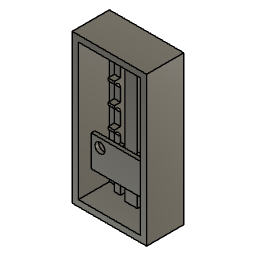
Progetto locker v3 (Autodesk Fusion 360 design; units mm, degrees)
Autodesk Fusion 360 part; units mm, degrees
note: some values were not read from the file. Chosen so that the rebuilt part matches the saved one: where a step ends.
sketch "Schizzo1" plane through (0, 0, 0) normal (0, 1, 0) x (1, 0, 0) in component "Scatola di fissaggio"
  line L0 (-30, -60) -> (30, -60)
  line L1 (30, -60) -> (30, 60)
  line L2 (30, 60) -> (-30, 60)
  line L3 (-30, 60) -> (-30, -60)
  point P0 (0, -60)
  point P1 (-30, 0)
  dimension "d1" = 60
  dimension "d2" = 120
  constraint horizontal L0
  constraint vertical L1
  constraint horizontal L2
  constraint vertical L3
  constraint midpoint L0 P0
  constraint midpoint L3 P1
  constraint vertical origin P0
  constraint horizontal origin P1
  measures "d1" distance of L0.start L0.end
  measures "d2" distance of L0.start L2.end
extrude "Estrusione1" add sketch "Schizzo1" along normal blind 30 makes body 1 in component "Scatola di fissaggio"
shell "Svuotamento1" thickness 5 removed faces 1 at (-10, 0, 20) on bodies 1 in component "Scatola di fissaggio"
ref_plane "Piano di lavoro1" through (0, 12.5, -55) normal (0, 0, 1) x (1, 0, 0) in component "Guida lineare"
sketch "Schizzo1 (2)" plane through (0, 12.5, -55) normal (0, 0, 1) x (1, 0, 0) in component "Guida lineare"
  line L0 (0, -21.6959) -> (0, 27.9147) construction
  line L1 (0, 5) -> (-5, 5)
  line L2 (-5, 5) -> (-5, 8.5)
  line L3 (-3.5, 10) -> (-2.5, 10)
  line L4 (-2.5, 10) -> (-2.5, 12.5)
  line L5 (25, 12.5) -> (-25, 12.5)
  line L6 (-5, 8.5) -> (-3.5, 10)
  line L7 (0, 5) -> (5, 5)
  line L8 (5, 5) -> (5, 8.5)
  line L9 (5, 8.5) -> (3.5, 10)
  line L10 (3.5, 10) -> (2.5, 10)
  line L11 (2.5, 10) -> (2.5, 12.5)
  point P0 (-5, 10)
  dimension "d7" = 2.5
  dimension "d8" = 5
  dimension "d9" = 5
  dimension "d10" = 2.5
  dimension "d11" = 1.5
  dimension "d12" = 1.5
  constraint vertical L0
  constraint coincident origin L0
  constraint coincident L0 L1.start
  constraint perpendicular L0 L1
  constraint perpendicular L1 L2
  constraint perpendicular L2 L3
  constraint perpendicular L3 L4
  constraint coincident L4.end L5
  constraint coincident P0 L2
  constraint coincident P0 L3
  constraint symmetric L0 L1.start L7.start
  constraint symmetric L0 L1.end L7.end
  constraint symmetric L0 L3.end L10.end
  constraint symmetric L0 L4.end L11.end
  constraint symmetric L0 L2.end L8.end
  constraint symmetric L0 L3.start L9.end
  measures "d7" distance of L3.end L4.end
  measures "d8" distance of L1.end P0
  measures "d9" distance of L1.start L1.end
  measures "d10" distance of L0 L4
  measures "d11" distance of P0 L2.end
  measures "d12" distance of P0 L3.start
extrude "Estrusione1'" add sketch "Schizzo1 (2)" along normal blind 110 separate body makes body 2 in component "Guida lineare"
sketch "Schizzo5" plane through (0, 0, 0) normal (0, 0, 1) x (1, 0, 0) in component "Base mobile"
  line L0 (5, 21) -> (3.5, 22.5)
  line L1 (5, 17.5) -> (5, 21)
  line L2 (0, 17.5) -> (5, 17.5)
  line L3 (0, 17) -> (5.5, 17)
  line L4 (5.5, 17) -> (5.5, 21.2071)
  line L5 (5.5, 21.2071) -> (3.8536, 22.8536)
  line L6 (3.8536, 22.8536) -> (8.8536, 22.8536)
  line L7 (8.8536, 22.8536) -> (8.8536, 12.8536)
  line L8 (8.8536, 12.8536) -> (0, 12.8536)
  line L9 (0, -9.1959) -> (0, 40.4147)
  line L10 (-8.8536, 12.8536) -> (0, 12.8536)
  line L11 (-8.8536, 22.8536) -> (-8.8536, 12.8536)
  line L12 (0, 17) -> (-5.5, 17)
  line L13 (-5.5, 17) -> (-5.5, 21.2071)
  line L14 (-3.8536, 22.8536) -> (-8.8536, 22.8536)
  line L15 (-5.5, 21.2071) -> (-3.8536, 22.8536)
  dimension "d24" = 0.5
  dimension "d25" = 10
  dimension "d26" = 5
  constraint perpendicular L1 L6
  constraint perpendicular L6 L7
  constraint perpendicular L7 L8
  constraint coincident L8.end L9
  constraint symmetric L3.start L9 L12.start
  constraint symmetric L3.end L9 L12.end
  constraint symmetric L4.end L9 L13.end
  constraint symmetric L5.end L9 L14.start
  constraint symmetric L6.end L9 L11.start
  constraint symmetric L7.end L9 L10.start
  constraint symmetric L8.end L9 L10.end
  measures "d25" distance of L6.end L7.end
  measures "d26" distance of L5.end L6.end
extrude "Estrusione2" add sketch "Schizzo5" along normal blind 5 and the other way blind 5 separate body makes body 3 in component "Base mobile"
sketch "Schizzo6" plane through (0, 12.8536, 0) normal (0, -1, 0) x (1, 0, 0) in component "Base mobile"
  line L0 (8.8536, -5) -> (8.8536, 5)
  line L1 (8.8536, 5) -> (-8.8536, 5)
  line L2 (-8.8536, 5) -> (-8.8536, -5)
  line L3 (-8.8536, -5) -> (8.8536, -5)
  line L4 (20, -12.5) -> (-20, -12.5)
  line L5 (-20, -12.5) -> (-20, 12.5)
  line L6 (-20, 12.5) -> (20, 12.5)
  line L7 (20, 12.5) -> (20, -12.5)
  point P0 (0, -12.5)
  point P1 (20, 0)
  dimension "d31" = 40
  dimension "d32" = 25
  constraint horizontal L4
  constraint vertical L5
  constraint horizontal L6
  constraint vertical L7
  constraint midpoint L4 P0
  constraint midpoint L7 P1
  constraint horizontal origin P1
  constraint vertical origin P0
  measures "d31" distance of L4.start L4.end
  measures "d32" distance of L4.start L6.end
extrude "Estrusione3" add sketch "Schizzo6" along normal blind 3 separate body contours L0 L1 L2 L3 | L4 L5 L6 L7 makes body 4 in component "Base mobile"
sketch "Schizzo1 (3)" plane through (0, 25, 0) normal (0, -1, 0) x (1, 0, 0) in component "cremagliera"
  line L0 (-25, 55) -> (-25, -55)
  line L1 (-25, -55) -> (25, -55)
  line L2 (25, -55) -> (25, 55)
  line L3 (25, 55) -> (-25, 55)
  line L4 (-11, -55) -> (-16, -55)
  line L5 (-16, -55) -> (-16, 55)
  line L6 (-16, 55) -> (-11, 55)
  line L7 (-11, 55) -> (-11, -55)
  dimension "d35" = 5
  dimension "d36" = 11
  constraint horizontal L4
  constraint vertical L5
  constraint horizontal L6
  constraint vertical L7
  constraint collinear L1 L4
  constraint collinear L3 L6
  measures "d35" distance of L4.start L4.end
  measures "d36" distance of origin L7
extrude "Estrusione1''" add sketch "Schizzo1 (3)" along normal blind 10 separate body contours L1 L3 L4 L5 L6 L7 makes body 5 in component "cremagliera"
sketch "Schizzo7" plane through (0, 9.8536, 0) normal (0, -1, 0) x (1, 0, 0) in component "Base mobile"
  line L0 (20, 12.5) -> (-20, 12.5)
  line L1 (-20, 12.5) -> (-20, -12.5)
  line L2 (-20, -12.5) -> (20, -12.5)
  line L3 (20, -12.5) -> (20, 12.5)
  circle A0 centre (-13, 5.5) radius 4
  dimension "d51" = 8
  dimension "d53" = 7
  dimension "d54" = 7
  measures "d51" diameter of A0
  measures "d53" distance of L0 A0.centre
  measures "d54" distance of L1 A0.centre
extrude "Estrusione4" cut sketch "Schizzo7" along normal up to far side of body 4 contours A0 bodies 4 in component "Base mobile"
sketch "Schizzo3" plane through (-16, 0, 0) normal (-1, 0, 0) x (0, -1, 0) in component "cremagliera"
  line L0 (-25, 55) -> (-25, -55)
  line L1 (-25, -55) -> (-15, -55)
  line L2 (-15, -55) -> (-15, 55)
  line L3 (-15, 55) -> (-25, 55)
  arc A0 (-15, -26) -> (-20, -31) centre (-15, -31) ccw
  line L4 (-20, -77.8463) -> (-20, -55) construction
  line L5 (-20, -31) -> (-20, 61.2431) construction
  line L6 (-15, -26) -> (-15, -24)
  line L7 (-20, -24) -> (-20, -14)
  line L8 (-15, -24) -> (-20, -24)
  arc A1 (-15, -9) -> (-20, -14) centre (-15, -14) ccw
  line L9 (-15, -9) -> (-15, -7)
  line L10 (-15, -7) -> (-20, -7)
  line L11 (-20, -7) -> (-20, 3)
  arc A2 (-15, 8) -> (-20, 3) centre (-15, 3) ccw
  line L12 (-15, 8) -> (-15, 10)
  line L13 (-20, 10) -> (-15, 10)
  line L14 (-20, 10) -> (-20, 20)
  arc A3 (-15, 25) -> (-20, 19.9924) centre (-15, 20) ccw
  line L15 (-15, 25) -> (-15, 27)
  line L16 (-20, 27) -> (-15, 27)
  line L17 (-20, 27) -> (-20, 37)
  arc A4 (-15, 42) -> (-20, 37) centre (-15, 37) ccw
  line L18 (-15, 42) -> (-15, 44)
  line L19 (-20, 44) -> (-20, 55)
  line L20 (-15, 44) -> (-20, 44)
  line L21 (-20, -31) -> (-20, -55)
  dimension "d57" = 5
  dimension "d58" = 24
  dimension "d59" = 2
  dimension "d60" = 10
  dimension "d61" = 2
  dimension "d62" = 10
  dimension "d63" = 2
  dimension "d64" = 10
  dimension "d65" = 2
  dimension "d66" = 10
  dimension "d67" = 2
  constraint parallel L0 L4
  constraint coincident L2 A0.centre
  constraint tangent A0 L4
  constraint midpoint L1 L4.end
  constraint coincident L2 A0.start
  constraint collinear L4 L5
  constraint coincident L2 L6.end
  constraint parallel L2 L6
  constraint coincident L5 L7.start
  constraint coincident L5 L7.end
  constraint perpendicular L7 L8
  constraint coincident L2 A1.centre
  constraint horizontal L7.end A1.centre
  constraint coincident L2 A1.start
  constraint coincident L2 L9.end
  constraint coincident L5 L10.end
  constraint perpendicular L5 L10
  constraint coincident L5 L11.end
  constraint coincident L2 A2.centre
  constraint horizontal L11.end A2.centre
  constraint coincident L2 A2.start
  constraint coincident L2 L12.end
  constraint parallel L2 L12
  constraint coincident L5 L13.start
  constraint perpendicular L2 L13
  constraint coincident L5 L14.end
  constraint coincident L2 A3.centre
  constraint coincident L14.end A3
  constraint horizontal L14.end A3.centre
  constraint coincident L2 A3.start
  constraint coincident L5 A3.end
  constraint coincident L2 L15.end
  constraint coincident L5 L16.start
  constraint coincident L5 L17.end
  constraint horizontal L16
  constraint coincident L2 A4.centre
  constraint tangent L17 A4
  constraint coincident L2 A4.start
  constraint coincident L2 L18.end
  constraint parallel L2 L18
  constraint coincident L5 L19.start
  constraint midpoint L3 L19.end
  constraint perpendicular L3 L19
  constraint perpendicular L19 L20
  measures "d57" distance of L0 L4
  measures "d58" distance of L1.end A0.centre
  measures "d59" distance of A0.start L6.end
  measures "d60" distance of L7.start L7.end
  measures "d61" distance of A1.start L9.end
  measures "d62" distance of L10.end L11.end
  measures "d63" distance of A2.start L12.end
  measures "d64" distance of L13.start L14.end
  measures "d65" distance of A3.start L15.end
  measures "d66" distance of L16.start L17.end
  measures "d67" distance of A4.start L18.end
extrude "Estrusione3'" cut sketch "Schizzo3" against normal up to surface (5 mm away) contours L2 L3 L19 L20 | L1 L2 A0 L21 | L2 L16 L17 A4 | L2 L7 L8 A1 | L2 L13 L14 A3 | L2 L10 L11 A2 bodies 5 in component "cremagliera"
sketch "Schizzo4" plane through (0, 20, 0) normal (0, -1, 0) x (1, 0, 0) in component "cremagliera"
  line L0 (-11, -55) -> (-11, -31)
  line L1 (-11, -31) -> (-16, -31)
  line L2 (-16, -31) -> (-16, -55)
  line L3 (-16, -55) -> (-11, -55)
  circle A0 centre (-13.5, -45) radius 2
  circle A1 centre (-13.5, 50) radius 2
  line L4 (-16, 44) -> (-16, 55)
  line L5 (-25, 55) -> (25, 55)
  dimension "d70" = 4
  dimension "d71" = 2.5
  dimension "d72" = 10
  dimension "d73" = 4
  dimension "d74" = 2.5
  dimension "d75" = 5
  measures "d70" diameter of A0
  measures "d71" distance of L2 A0.centre
  measures "d72" distance of L3 A0.centre
  measures "d73" diameter of A1
  measures "d74" distance of A1.centre L4
  measures "d75" distance of A1.centre L5
extrude "Estrusione4'" cut sketch "Schizzo4" against normal up to surface (5 mm away) contours A0 | A1 bodies 5 in component "cremagliera"
sketch "Schizzo2" plane through (0, 0, 0) normal (0, 1, 0) x (1, 0, 0) in component "Scatola di fissaggio"
  circle A0 centre (-13.5, 45) radius 2
  circle A1 centre (-13.5, -50) radius 2
extrude "Estrusione2'" cut sketch "Schizzo2" along normal up to surface (30 mm away) bodies 1 in component "Scatola di fissaggio"
component "Scatola di fissaggio" placed x (1, 0, 0) y (0, 1, 0) z (0, 0, 1) at (0, 0, 0)
component "Guida lineare" placed x (1, 0, 0) y (0, 1, 0) z (0, 0, 1) at (0, 0, 0)
component "Base mobile" placed x (1, 0, 0) y (0, 1, 0) z (0, 0, 1) at (0, 0, 0)
component "cremagliera" placed x (1, 0, 0) y (0, 1, 0) z (0, 0, 1) at (0, 0, 0)
equation "d12 = d11"
